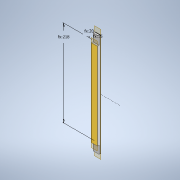
# Autodesk Inventor part: spacer_no_wireholder
Saved by Autodesk Inventor 2020 (Build 240168000, 168)
## iProperties
Created: 2021-01-31
Part Number: spacer_no_wireholder
Material: Generic
Document SubType Name: Modeling
Designer: phamv
Density: 1 g/cm^3
Appearance: Default
Author: phamv
Autodesk Inventor part; units mm, degrees
ref_plane "YZ Plane" through (0, 0, 0) normal (1, 0, 0) x (0, 1, 0)
ref_plane "XZ Plane" through (0, 0, 0) normal (0, 1, 0) x (-1, 0, 0)
sketch "Sketch1" plane through (0, 0, 0) normal (0, 0, 1) x (1, 0, 0)
  line L0 (0, 109) -> (15, 109)
  line L1 (15, 109) -> (15, -109)
  line L2 (15, -109) -> (0, -109)
  line L3 (0, -109) -> (0, 109)
  line L4 (0, 109) -> (15, 109)
  line L5 (15, 109) -> (15, 129)
  line L6 (15, 129) -> (0, 129)
  line L7 (0, 129) -> (0, 109)
  line L8 (0, 0) -> (65.2532, 0) construction
  line L9 (15, -109) -> (15, -129)
  line L10 (15, -129) -> (0, -129)
  line L11 (0, -129) -> (0, -109)
  dimension "d0" = 218
  dimension "d1" = 15
  dimension "d3" = 20
  constraints: 24 end point, 4 parallel, 3 horizontal, 3 symmetric about line, 2 perpendicular, 1 coincident, 1 collinear, 1 midpoint
  measures "d0" distance between parallel lines of L2 L0
  measures "d1" distance between parallel lines of L1 L3
  measures "d3" distance between parallel lines of L0 L6
extrude "Extrusion1" add sketch "Sketch1" along normal blind 8 contours L0 L1 L2 L3
extrude "Extrusion2" add sketch "Sketch1" along normal blind 4 contours L7 L6 L5 L0 | L2 L9 L10 L11
ref_plane "spacer_surface Plane" through (0, 0, 8) normal (0, 0, 1) x (1, 0, 0)
sketch "Sketch2" plane through (0, 0, 8) normal (0, 0, 1) x (1, 0, 0)
  line L0 (0, 8) -> (15, 8)
  line L1 (15, 8) -> (15, 2)
  line L2 (15, 2) -> (0, 2)
  line L3 (0, 2) -> (0, 8)
  line L4 (0, 109) -> (0, -109) projected
  line L5 (15, -109) -> (15, 109) projected
  line L6 (0, 0) -> (65.2532, 0) construction
  line L7 (0, 129) -> (0, -129) projected
  line L8 (0, 3) -> (15, 3)
  line L9 (0, 7) -> (15, 7)
  point P0 (0, 5)
  point P1 (15, 5)
  point P2 (0, 3)
  point P3 (0, 7)
  dimension "d0" = 218
  dimension "d12" = 1
  dimension "d13" = 1
  dimension "d14" = 4
  dimension "d15" = 2
  constraints: 12 end point, 5 point on line, 3 perpendicular, 2 midpoint, 2 parallel, 1 horizontal, 2 other
  measures "d12" distance between parallel lines of L9 L0
  measures "d13" distance between parallel lines of L2 L8
  measures "d14" distance between parallel lines of L8 L9
  measures "d15" distance between parallel lines of L2 L6
extrude "Extrusion3" [suppressed]
pattern_linear "Rectangular Pattern1" [suppressed]
mirror "Mirror1" [suppressed]
equation "\"d0\" = spacer_length"
equation "\"d1\" = spacer_width"
equation "\"d3\" = lock_length"
equation "\"d4\" = spacer_height"
equation "\"d6\" = lock_height"
equation "\"d12\" = holder_thickness"
equation "\"d13\" = holder_thickness"
equation "\"d14\" = wire_diameter"
equation "\"d15\" = 0.5 * wire_diameter"
equation "\"d16\" = wire_diameter"
equation "\"spacer_length\" = 218"
equation "\"spacer_width\" = 15"
equation "\"spacer_height\" = 8"
equation "\"lock_length\" = 20"
equation "\"lock_height\" = 4"
equation "\"wire_diameter\" = 4"
equation "\"wire_holder_offset\" = 0.1"
equation "\"holder_thickness\" = 1"
body "Solid1"
